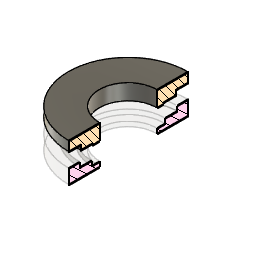
Waveplate size adapter (Autodesk Fusion 360 design; units mm, degrees)
Autodesk Fusion 360 part; units mm, degrees
sketch "Sketch1" plane through (0, 0, 0) normal (0, 0, 1) x (1, 0, 0) in component "Base"
  circle A0 centre (0, 0) radius 12.5
  circle A1 centre (0, 0) radius 6
  dimension "d38" = 25
  dimension "d39" = 12
  constraint coincident A0.centre A1.centre
  constraint concentric A0 A1
  measures "d38" diameter of A0
  measures "d39" diameter of A1
extrude "Extrude1" add sketch "Sketch1" along normal blind 3 makes body 1 in component "Base"
sketch "Sketch2" plane through (0, 0, 3) normal (0, 0, 1) x (-1, 0, 0) in component "Base"
  circle A0 centre (0, 0) radius 6
  circle A1 centre (0, 0) radius 12.5
  circle A2 centre (0, 0) radius 10.2
  dimension "d44" = 20.4
  constraint coincident A0.centre A1.centre
  measures "d44" diameter of A2
extrude "Extrude2" cut sketch "Sketch2" against normal blind 1 contours A2 bodies 1 in component "Base"
sketch "Sketch3" plane through (0, 0, 2) normal (0, 0, 1) x (-1, 0, 0) in component "Base"
  circle A0 centre (0, 0) radius 6
  circle A1 centre (0, 0) radius 10.2
  circle A2 centre (0, 0) radius 7.7
  dimension "d48" = 15.4
  constraint coincident A0.centre A1.centre
  measures "d48" diameter of A2
extrude "Extrude3" cut sketch "Sketch3" against normal blind 1 contours A2 bodies 1 in component "Base"
sketch "Sketch1 (2)" plane through (0, 0, 0) normal (0, 0, 1) x (1, 0, 0) in component "Lid"
  circle A0 centre (0, 0) radius 7.5
  circle A1 centre (0, 0) radius 6
  dimension "d51" = 12
  dimension "d52" = 15
  constraint coincident A0.centre A1.centre
  constraint concentric A0 A1
  measures "d51" diameter of A1
  measures "d52" diameter of A0
extrude "Extrude1'" add sketch "Sketch1 (2)" along normal blind 0.3 separate body makes body 2 in component "Lid"
sketch "Sketch2 (2)" plane through (0, 0, 0.3) normal (0, 0, 1) x (-1, 0, 0) in component "Lid"
  circle A0 centre (0, 0) radius 6
  circle A1 centre (0, 0) radius 7.5
  circle A2 centre (0, 0) radius 6
  circle A3 centre (0, 0) radius 10
  dimension "d55" = 12
  dimension "d56" = 20
  constraint coincident A0.centre A1.centre
  constraint concentric A2 A3
  measures "d55" diameter of A2
  measures "d56" diameter of A3
extrude "Extrude2'" add sketch "Sketch2 (2)" along normal blind 1 contours A1 | A3 bodies 2 in component "Lid"
sketch "Sketch3 (2)" plane through (0, 0, 1.3) normal (0, 0, 1) x (-1, 0, 0) in component "Lid"
  circle A0 centre (0, 0) radius 6
  circle A1 centre (0, 0) radius 10
  circle A2 centre (0, 0) radius 6
  circle A3 centre (0, 0) radius 12.5
  dimension "d59" = 25
  dimension "d60" = 12
  constraint coincident A0.centre A1.centre
  constraint concentric A2 A3
  measures "d59" diameter of A3
  measures "d60" diameter of A2
extrude "Extrude3'" add sketch "Sketch3 (2)" along normal blind 2 contours A1 | A3 bodies 2 in component "Lid"
component "Base" placed x (1, 0, 0) y (0, 1, 0) z (0, 0, 1) at (0, 0, 0)
component "Lid" placed x (1, 0, 0) y (0, 1, 0) z (0, 0, 1) at (0, 0, 0)
equation "waveplate_t = 1 mm"
equation "waveplate_d = 15 mm"
equation "clear_aperture = 12 mm"
equation "external_d = 25 mm"
equation "pressure_extension = 0.3 mm"
equation "margin = 0.2 mm"
equation "mid_ring_d = 20 mm"
equation "d39 = clear_aperture"
equation "lid_external_t = 2 mm"
equation "base_t = 3 mm"
equation "d42 = base_t"
equation "d44 = mid_ring_d + 2 * margin"
equation "lid_insert_t = 1 mm"
equation "d46 = -lid_insert_t"
equation "d48 = waveplate_d + 2 * margin"
equation "d49 = -waveplate_t"
equation "d51 = clear_aperture"
equation "d52 = waveplate_d"
equation "d53 = pressure_extension"
equation "d55 = clear_aperture"
equation "d56 = mid_ring_d"
equation "d57 = lid_insert_t"
equation "d59 = external_d"
equation "d60 = clear_aperture"
equation "d61 = lid_external_t"
